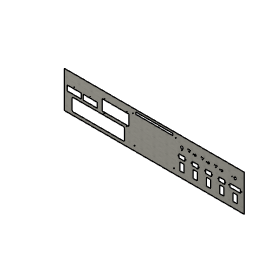
002_mounting_plate (Autodesk Fusion 360 design; units mm, degrees)
Autodesk Fusion 360 part; units mm, degrees
note: some values were not read from the file. Set by a fixed rule: the direction of a hole.
sketch "Sketch1" plane through (360, 70, -13) normal (0, 0, -1) x (1, 0, 0)
  line L0 (100, 7.5) -> (124, 7.5)
  line L1 (124, 7.5) -> (124, -7.5)
  line L2 (124, -7.5) -> (100, -7.5)
  line L3 (100, -7.5) -> (100, 7.5)
  circle A0 centre (274, -35) radius 3.5
  circle A1 centre (220, -35) radius 3.5
  circle A2 centre (220, 35) radius 6.5
  circle A3 centre (166, 35) radius 6.5
  circle A4 centre (112, 35) radius 6.5
  circle A5 centre (274, 35) radius 6.5
  circle A6 centre (328, 35) radius 6.5
  line L4 (-210, -3.5) -> (-105, -3.5) construction
  line L5 (-105, -3.5) -> (-105, -43.5) construction
  line L6 (-105, -43.5) -> (-210, -43.5) construction
  line L7 (-210, -43.5) -> (-210, -3.5) construction
  circle A7 centre (328, -35) radius 4.5
  arc A8 (-121, 55.5) -> (-126, 60.5) centre (-126, 55.5) ccw
  line L8 (-121, 55.5) -> (-121, 14.5)
  arc A9 (-126, 9.5) -> (-121, 14.5) centre (-126, 14.5) ccw
  line L9 (-126, 9.5) -> (-329, 9.5)
  arc A10 (-334, 14.5) -> (-329, 9.5) centre (-329, 14.5) ccw
  line L10 (-334, 14.5) -> (-334, 55.5)
  arc A11 (-329, 60.5) -> (-334, 55.5) centre (-329, 55.5) ccw
  line L11 (-329, 60.5) -> (-126, 60.5)
  circle A12 centre (166, -35) radius 3.5
  circle A13 centre (112, -35) radius 5
  line L12 (-360, 70) -> (-360, -70)
  line L13 (-360, -70) -> (360, -70)
  line L14 (360, -70) -> (360, 70)
  line L15 (360, 70) -> (-360, 70)
  line L16 (-333.4, -12.9) -> (-333.4, -4.4) construction
  line L17 (-297.4, -2.4) -> (-352.4, -2.4) construction
  line L18 (-352.4, -2.4) -> (-352.4, -50.4) construction
  line L19 (-352.4, -50.4) -> (-297.4, -50.4) construction
  line L20 (-297.4, -50.4) -> (-297.4, -2.4) construction
  line L21 (-316.4, -4.4) -> (-316.4, -12.9) construction
  line L22 (-333.4, -4.4) -> (-333.4, -12.9) construction
  line L23 (-316.4, -12.9) -> (-316.4, -4.4) construction
  line L24 (-268.6, -4.4) -> (-268.6, -12.9) construction
  line L25 (-251.6, -12.9) -> (-251.6, -4.4) construction
  line L26 (-251.6, -4.4) -> (-251.6, -12.9) construction
  line L27 (-268.6, -12.9) -> (-268.6, -4.4) construction
  line L28 (-232.6, -2.4) -> (-287.6, -2.4) construction
  line L29 (-287.6, -2.4) -> (-287.6, -50.4) construction
  line L30 (-287.6, -50.4) -> (-232.6, -50.4) construction
  line L31 (-232.6, -50.4) -> (-232.6, -2.4) construction
  line L32 (-231.6, -22.4) -> (-288.6, -22.4)
  line L33 (-288.6, -22.4) -> (-288.6, -1.4)
  line L34 (-288.6, -1.4) -> (-231.6, -1.4)
  line L35 (-231.6, -1.4) -> (-231.6, -22.4)
  line L36 (-287.6, -26.4) -> (-297.4, -26.4) construction
  line L37 (-292.5, -26.4) -> (-292.5, -42) construction
  line L38 (-353.4, -22.4) -> (-296.4, -22.4)
  line L39 (-353.4, -1.4) -> (-353.4, -22.4)
  line L40 (-296.4, -1.4) -> (-353.4, -1.4)
  line L41 (-296.4, -22.4) -> (-296.4, -1.4)
  line L42 (232, -7.5) -> (208, -7.5)
  line L43 (208, -7.5) -> (208, 7.5)
  line L44 (208, 7.5) -> (232, 7.5)
  line L45 (232, 7.5) -> (232, -7.5)
  line L46 (178, -7.5) -> (154, -7.5)
  line L47 (154, -7.5) -> (154, 7.5)
  line L48 (154, 7.5) -> (178, 7.5)
  line L49 (178, 7.5) -> (178, -7.5)
  line L50 (286, -7.5) -> (262, -7.5)
  line L51 (262, -7.5) -> (262, 7.5)
  line L52 (262, 7.5) -> (286, 7.5)
  line L53 (286, 7.5) -> (286, -7.5)
  circle A14 centre (328, 0) radius 4.6 construction
  circle A15 centre (343, 0) radius 4.6 construction
  circle A16 centre (313, 0) radius 4.6 construction
  line L54 (307, -7) -> (349, -7)
  line L55 (349, -7) -> (349, 7)
  line L56 (349, 7) -> (307, 7)
  line L57 (307, 7) -> (307, -7)
  line L58 (328, 0) -> (328, -7) construction
  line L59 (349, 0) -> (360, 0) construction
  circle A17 centre (353, 0) radius 1.6
  circle A18 centre (303, 0) radius 1.6
  line L60 (-360, 0) -> (360, 0) construction
  line L61 (0, -70) -> (0, 70) construction
  line L62 (-235, -43.5) -> (-285, -43.5) construction
  line L63 (-285, -43.5) -> (-285, -13.5) construction
  line L64 (-285, -13.5) -> (-235, -13.5) construction
  line L65 (-235, -13.5) -> (-235, -43.5) construction
  circle A19 centre (-260, -28.5) radius 2
  line L66 (-260, -43.5) -> (-260, -28.5) construction
  line L67 (-260, -28.5) -> (-235, -28.5) construction
  circle A20 centre (-325, -28.5) radius 2
  arc A21 (-333.4, -12.9) -> (-316.4, -12.9) centre (-324.9, -12.9) ccw
  line L68 (-333.4, -4.4) -> (-316.4, -4.4)
  line L69 (-316.4, -4.4) -> (-333.4, -4.4)
  arc A22 (-333.4, -12.9) -> (-316.4, -12.9) centre (-324.9, -12.9) ccw
  line L70 (-251.6, -4.4) -> (-268.6, -4.4)
  arc A23 (-268.6, -12.9) -> (-251.6, -12.9) centre (-260.1, -12.9) ccw
  line L71 (-268.6, -4.4) -> (-251.6, -4.4)
  arc A24 (-268.6, -12.9) -> (-251.6, -12.9) centre (-260.1, -12.9) ccw
  line L72 (-231.6, -21.4) -> (-288.6, -21.4) construction
  line L73 (365, 73) -> (-365, 73)
  line L74 (-365, 73) -> (-365, -75)
  line L75 (-365, -75) -> (365, -75)
  line L76 (365, -75) -> (365, 73)
  dimension "d326" = 42
  dimension "d327" = 14
  dimension "d330" = 3.2
  dimension "d331" = 7
  dimension "d334" = 4
  dimension "d811" = 4
  dimension "d819" = 1
  dimension "d820" = 1
  dimension "d821" = 1
  dimension "d822" = 1
  constraint horizontal L32
  constraint vertical L33
  constraint horizontal L34
  constraint vertical L35
  constraint midpoint L29 L36.start
  constraint midpoint L20 L36.end
  constraint midpoint L36 L37.start
  constraint perpendicular L36 L37
  constraint symmetric L32.start L37 L38.start
  constraint symmetric L32.end L37 L38.end
  constraint symmetric L33.end L37 L40.start
  constraint symmetric L34.end L37 L39.start
  constraint horizontal L54
  constraint vertical L55
  constraint horizontal L56
  constraint vertical L57
  constraint coincident A14.centre L58.start
  constraint midpoint L54 L58.end
  constraint vertical L58
  constraint midpoint L55 L59.start
  constraint midpoint L14 L59.end
  constraint horizontal L59
  constraint symmetric L58 A17 A18
  constraint midpoint L12 L60.start
  constraint midpoint L13 L61.start
  constraint midpoint L15 L61.end
  constraint midpoint L62 L66.start
  constraint coincident A19.centre L66.end
  constraint perpendicular L62 L66
  constraint midpoint L65 L67.end
  constraint perpendicular L65 L67
  constraint symmetric L37 A19 A20
  constraint coincident L35 L72.start
  constraint coincident L33 L72.end
  constraint perpendicular L33 L72
  constraint tangent A23 L72
  measures "d326" distance of L54.start L54.end
  measures "d327" distance of L54.start L56.end
  measures "d330" diameter of A17
  measures "d331" distance of L54 A17.centre
  measures "d334" distance of L55 A17.centre
  measures "d811" diameter of A19
  measures "d819" distance of L32 L72
  measures "d820" distance of L31 L35
  measures "d821" distance of L28 L34
  measures "d822" distance of L29 L33
extrude "Extrude1" add sketch "Sketch1" along normal blind 1 contours A2 | A3 | A4 | A5 | A6 | L12 L13 L14 L15 | A17 | A18 | A19 | A20
sketch "Sketch3" plane through (0, 0, -14) normal (0, 0, -1) x (-1, 0, 0)
  circle A0 centre (-580, 105) radius 3.5
  circle A1 centre (-634, 105) radius 3.5
  line L0 (-484, 77.5) -> (-460, 77.5)
  line L1 (-460, 77.5) -> (-460, 62.5)
  line L2 (-460, 62.5) -> (-484, 62.5)
  line L3 (-484, 62.5) -> (-484, 77.5)
  line L4 (-622, 62.5) -> (-646, 62.5)
  line L5 (-646, 62.5) -> (-646, 77.5)
  line L6 (-646, 77.5) -> (-622, 77.5)
  line L7 (-622, 77.5) -> (-622, 62.5)
  circle A2 centre (-688, 105) radius 4.5
  line L8 (-514, 62.5) -> (-538, 62.5)
  line L9 (-538, 62.5) -> (-538, 77.5)
  line L10 (-538, 77.5) -> (-514, 77.5)
  line L11 (-514, 77.5) -> (-514, 62.5)
  line L12 (-568, 62.5) -> (-592, 62.5)
  line L13 (-592, 62.5) -> (-592, 77.5)
  line L14 (-592, 77.5) -> (-568, 77.5)
  line L15 (-568, 77.5) -> (-568, 62.5)
  arc A3 (-26, 55.5) -> (-31, 60.5) centre (-31, 55.5) ccw
  line L16 (-26, 55.5) -> (-26, 14.5)
  arc A4 (-31, 9.5) -> (-26, 14.5) centre (-31, 14.5) ccw
  line L17 (-31, 9.5) -> (-234, 9.5)
  arc A5 (-239, 14.5) -> (-234, 9.5) centre (-234, 14.5) ccw construction
  line L18 (-239, 14.5) -> (-239, 55.5) construction
  arc A6 (-234, 60.5) -> (-239, 55.5) centre (-234, 55.5) ccw construction
  line L19 (-234, 60.5) -> (-31, 60.5)
  line L20 (-667, 77) -> (-667, 63)
  line L21 (-667, 63) -> (-709, 63)
  line L22 (-709, 63) -> (-709, 77)
  line L23 (-709, 77) -> (-667, 77)
  line L24 (-63.6, 71.4) -> (-63.6, 92.4)
  line L25 (-63.6, 92.4) -> (-6.6, 92.4)
  line L26 (-6.6, 92.4) -> (-6.6, 71.4)
  line L27 (-6.6, 71.4) -> (-63.6, 71.4)
  circle A7 centre (-526, 105) radius 3.5
  circle A8 centre (-472, 105) radius 5
  line L28 (-71.4, 71.4) -> (-128.4, 71.4)
  line L29 (-128.4, 71.4) -> (-128.4, 92.4)
  line L30 (-128.4, 92.4) -> (-71.4, 92.4)
  line L31 (-71.4, 92.4) -> (-71.4, 71.4)
  line L32 (-720, 0) -> (0, 0)
  line L33 (0, 0) -> (0, 140)
  line L34 (0, 140) -> (-720, 140)
  line L35 (-720, 140) -> (-720, 0)
  line L36 (-275, 17.5) -> (-275, 128.5) construction
  line L37 (-445, 17.5) -> (-275, 17.5) construction
  line L38 (-445, 128.5) -> (-445, 17.5) construction
  line L39 (-275, 128.5) -> (-445, 128.5) construction
  circle A9 centre (-447, 126.5) radius 1.5
  line L40 (-275, 73) -> (-445, 73) construction
  line L41 (-360, 17.5) -> (-360, 128.5) construction
  circle A10 centre (-273, 126.5) radius 1.5
  circle A11 centre (-440, 16) radius 1.5
  circle A12 centre (-280, 16) radius 1.5
  line L42 (-285, 128.5) -> (-435, 128.5)
  line L43 (-435, 128.5) -> (-435, 136.5)
  line L44 (-435, 136.5) -> (-285, 136.5)
  line L45 (-285, 136.5) -> (-285, 128.5)
  line L46 (-200, 114.5) -> (-200, 113.5) construction
  line L47 (-200, 113.5) -> (-205, 113.5) construction
  line L48 (-205, 113.5) -> (-205, 114.5) construction
  line L49 (-205, 114.5) -> (-255, 114.5) construction
  line L50 (-255, 114.5) -> (-255, 96) construction
  line L51 (-255, 96) -> (-256, 96) construction
  line L52 (-256, 96) -> (-256, 91) construction
  line L53 (-256, 91) -> (-255, 91) construction
  line L54 (-255, 91) -> (-255, 72.5) construction
  line L55 (-255, 72.5) -> (-205, 72.5) construction
  line L56 (-205, 72.5) -> (-205, 73.5) construction
  line L57 (-205, 73.5) -> (-200, 73.5) construction
  line L58 (-200, 73.5) -> (-200, 72.5) construction
  line L59 (-200, 72.5) -> (-150, 72.5) construction
  line L60 (-150, 72.5) -> (-150, 91) construction
  line L61 (-150, 96) -> (-150, 114.5) construction
  line L62 (-150, 114.5) -> (-200, 114.5) construction
  line L63 (-256.5, 115) -> (-148.5, 115)
  line L64 (-148.5, 115) -> (-148.5, 72)
  line L65 (-148.5, 72) -> (-256.5, 72)
  line L66 (-256.5, 72) -> (-256.5, 115)
  line L67 (-150, 91) -> (-149, 91)
  line L68 (-149, 91) -> (-149, 96)
  line L69 (-149, 96) -> (-150, 96)
  dimension "d480" = 3
  dimension "d483" = 150
  dimension "d484" = 8
  dimension "d491" = 5
  dimension "d492" = 2
  dimension "d493" = 2
  dimension "d801" = 0.5
  dimension "d802" = 0.5
  dimension "d803" = 0.5
  constraint midpoint L36 L40.start
  constraint midpoint L38 L40.end
  constraint midpoint L37 L41.start
  constraint midpoint L39 L41.end
  constraint symmetric A9 L41 A10
  constraint horizontal L42
  constraint vertical L43
  constraint horizontal L44
  constraint vertical L45
  constraint coincident L39 L42.start
  constraint symmetric L41 L43 L45
  constraint equal A9 A11
  constraint equal A11 A12
  constraint symmetric L41 A11 A12
  constraint tangent L37 A11
  constraint horizontal L63
  constraint vertical L64
  constraint horizontal L65
  constraint vertical L66
  measures "d480" diameter of A9
  measures "d483" distance of L43.end L44.end
  measures "d484" distance of L42.end L43.end
  measures "d491" distance of L38 A11.centre
  measures "d492" distance of L39 A9.centre
  measures "d493" distance of L38 A9.centre
  measures "d801" distance of L59 L65
  measures "d802" distance of L52 L66
  measures "d803" distance of L49 L63
extrude "Extrude4" cut sketch "Sketch3" against normal up to surface (1 mm away) contours L42 L43 L44 L45 | L63 L64 L65 L66
hole "Hole1" at (447, 126.5, -14) at (440, 16, -14) at (280, 16, -14) at (273, 126.5, -14) direction (0, 0, 1) diameter 3.4 depth 2 tip angle 118
sketch "Sketch4" plane through (360, 70, -5) normal (0, 0, 1) x (1, 0, 0)
  circle A0 centre (146.55, 41.35) radius 1 construction
  circle A1 centre (141.55, 41.35) radius 1 construction
  circle A2 centre (136.55, 41.35) radius 1 construction
  circle A3 centre (141.55, 35) radius 1.5
  circle A4 centre (136.55, 41.35) radius 1.2
  circle A5 centre (141.55, 41.35) radius 1.2
  circle A6 centre (146.55, 41.35) radius 1.2
  circle A7 centre (141.55, 35) radius 1.6
  line L0 (158.5, 33.6282) -> (158.5, 36.2282) construction
  line L1 (158.5, 36.2282) -> (157.5, 36.2282) construction
  line L2 (157.5, 36.2282) -> (157.5, 33.6282) construction
  line L3 (157.5, 33.6282) -> (158.5, 33.6282) construction
  line L4 (157.3, 33.4282) -> (158.7, 33.4282)
  line L5 (158.7, 33.4282) -> (158.7, 36.4282)
  line L6 (158.7, 36.4282) -> (157.3, 36.4282)
  line L7 (157.3, 36.4282) -> (157.3, 33.4282)
  dimension "d578" = 0.2
  dimension "d579" = 0.2
  dimension "d580" = 0.2
  dimension "d581" = 3.2
  dimension "d628" = 0.2
  constraint concentric A3 A7
  measures "d581" diameter of A7
extrude "Extrude6" cut sketch "Sketch4" against normal up to surface (9 mm away) contours A5 | L4 L5 L6 L7
pattern_linear "R-Pattern1" count 3 spacing 54 along (1, 0, 0) of "Extrude6"
sketch "Sketch5" plane through (0, 0, -13) normal (0, 0, 1) x (1, 0, 0)
  circle A0 centre (609.55, 111.35) radius 1.2
  line L0 (625.3, 106.4282) -> (626.7, 106.4282)
  line L1 (626.7, 106.4282) -> (626.7, 103.4282)
  line L2 (626.7, 103.4282) -> (625.3, 103.4282)
  line L3 (625.3, 103.4282) -> (625.3, 106.4282)
  circle A1 centre (555.55, 111.35) radius 1.2
  line L4 (571.3, 106.4282) -> (572.7, 106.4282)
  line L5 (572.7, 106.4282) -> (572.7, 103.4282)
  line L6 (572.7, 103.4282) -> (571.3, 103.4282)
  line L7 (571.3, 103.4282) -> (571.3, 106.4282)
  circle A2 centre (501.55, 111.35) radius 1.2
  line L8 (517.3, 106.4282) -> (518.7, 106.4282)
  line L9 (518.7, 106.4282) -> (518.7, 103.4282)
  line L10 (518.7, 103.4282) -> (517.3, 103.4282)
  line L11 (517.3, 103.4282) -> (517.3, 106.4282)
  circle A3 centre (280, 16) radius 1.7
  circle A4 centre (447, 126.5) radius 1.7
  circle A5 centre (440, 16) radius 1.7
  circle A6 centre (273, 126.5) radius 1.7
  line L12 (285, 128.5) -> (285, 136.5)
  line L13 (285, 136.5) -> (435, 136.5)
  line L14 (435, 136.5) -> (435, 128.5)
  line L15 (435, 128.5) -> (285, 128.5)
  circle A7 centre (688, 105) radius 4.5
  arc A8 (31, 60.5) -> (26, 55.5) centre (31, 55.5) ccw
  line L16 (31, 60.5) -> (234, 60.5)
  arc A9 (239, 55.5) -> (234, 60.5) centre (234, 55.5) ccw
  line L17 (239, 55.5) -> (239, 14.5)
  arc A10 (234, 9.5) -> (239, 14.5) centre (234, 14.5) ccw
  line L18 (234, 9.5) -> (31, 9.5)
  arc A11 (26, 14.5) -> (31, 9.5) centre (31, 14.5) ccw
  line L19 (26, 14.5) -> (26, 55.5)
  line L20 (667, 63) -> (667, 77)
  line L21 (667, 77) -> (709, 77)
  line L22 (709, 77) -> (709, 63)
  line L23 (709, 63) -> (667, 63)
  line L24 (460, 77.5) -> (484, 77.5)
  line L25 (484, 77.5) -> (484, 62.5)
  line L26 (484, 62.5) -> (460, 62.5)
  line L27 (460, 62.5) -> (460, 77.5)
  line L28 (592, 62.5) -> (568, 62.5)
  line L29 (568, 62.5) -> (568, 77.5)
  line L30 (568, 77.5) -> (592, 77.5)
  line L31 (592, 77.5) -> (592, 62.5)
  circle A12 centre (580, 105) radius 3.5
  line L32 (646, 62.5) -> (622, 62.5)
  line L33 (622, 62.5) -> (622, 77.5)
  line L34 (622, 77.5) -> (646, 77.5)
  line L35 (646, 77.5) -> (646, 62.5)
  line L36 (63.6, 92.4) -> (63.6, 71.4)
  line L37 (63.6, 71.4) -> (6.6, 71.4)
  line L38 (6.6, 71.4) -> (6.6, 92.4)
  line L39 (6.6, 92.4) -> (63.6, 92.4)
  line L40 (538, 62.5) -> (514, 62.5)
  line L41 (514, 62.5) -> (514, 77.5)
  line L42 (514, 77.5) -> (538, 77.5)
  line L43 (538, 77.5) -> (538, 62.5)
  line L44 (128.4, 71.4) -> (71.4, 71.4)
  line L45 (71.4, 71.4) -> (71.4, 92.4)
  line L46 (71.4, 92.4) -> (128.4, 92.4)
  line L47 (128.4, 92.4) -> (128.4, 71.4)
  circle A13 centre (634, 105) radius 3.5
  circle A14 centre (472, 105) radius 5
  circle A15 centre (526, 105) radius 3.5
  line L48 (0, 0) -> (720, 0)
  line L49 (720, 0) -> (720, 140)
  line L50 (720, 140) -> (0, 140)
  line L51 (0, 140) -> (0, 0)
  circle A16 centre (457.625, 70) radius 1.5 construction
  circle A17 centre (486.375, 70) radius 1.5 construction
  circle A18 centre (457.625, 70) radius 1.7
  circle A19 centre (486.375, 70) radius 1.7
  line L52 (256.5, 115) -> (256.5, 72)
  line L53 (256.5, 72) -> (148.5, 72)
  line L54 (148.5, 72) -> (148.5, 115)
  line L55 (148.5, 115) -> (256.5, 115)
  dimension "d648" = 0.2
  constraint concentric A17 A19
  constraint equal A18 A19
sketch "Sketch6" plane through (0, 0, -13) normal (0, 0, 1) x (1, 0, 0)
  circle A0 centre (609.55, 111.35) radius 1.2
  line L0 (625.3, 106.4282) -> (626.7, 106.4282)
  line L1 (626.7, 106.4282) -> (626.7, 103.4282)
  line L2 (626.7, 103.4282) -> (625.3, 103.4282)
  line L3 (625.3, 103.4282) -> (625.3, 106.4282)
  circle A1 centre (555.55, 111.35) radius 1.2
  line L4 (571.3, 106.4282) -> (572.7, 106.4282)
  line L5 (572.7, 106.4282) -> (572.7, 103.4282)
  line L6 (572.7, 103.4282) -> (571.3, 103.4282)
  line L7 (571.3, 103.4282) -> (571.3, 106.4282)
  circle A2 centre (501.55, 111.35) radius 1.2
  line L8 (517.3, 106.4282) -> (518.7, 106.4282)
  line L9 (518.7, 106.4282) -> (518.7, 103.4282)
  line L10 (518.7, 103.4282) -> (517.3, 103.4282)
  line L11 (517.3, 103.4282) -> (517.3, 106.4282)
  circle A3 centre (280, 16) radius 1.7
  circle A4 centre (447, 126.5) radius 1.7
  circle A5 centre (440, 16) radius 1.7
  circle A6 centre (273, 126.5) radius 1.7
  line L12 (285, 128.5) -> (285, 136.5)
  line L13 (285, 136.5) -> (435, 136.5)
  line L14 (435, 136.5) -> (435, 128.5)
  line L15 (435, 128.5) -> (285, 128.5)
  line L16 (667, 63) -> (667, 77)
  line L17 (667, 77) -> (709, 77)
  line L18 (709, 77) -> (709, 63)
  line L19 (709, 63) -> (667, 63)
  circle A7 centre (634, 105) radius 3.5
  circle A8 centre (580, 105) radius 3.5
  line L20 (646, 62.5) -> (622, 62.5)
  line L21 (622, 62.5) -> (622, 77.5)
  line L22 (622, 77.5) -> (646, 77.5)
  line L23 (646, 77.5) -> (646, 62.5)
  line L24 (460, 77.5) -> (484, 77.5)
  line L25 (484, 77.5) -> (484, 62.5)
  line L26 (484, 62.5) -> (460, 62.5)
  line L27 (460, 62.5) -> (460, 77.5)
  line L28 (538, 62.5) -> (514, 62.5)
  line L29 (514, 62.5) -> (514, 77.5)
  line L30 (514, 77.5) -> (538, 77.5)
  line L31 (538, 77.5) -> (538, 62.5)
  line L32 (592, 62.5) -> (568, 62.5)
  line L33 (568, 62.5) -> (568, 77.5)
  line L34 (568, 77.5) -> (592, 77.5)
  line L35 (592, 77.5) -> (592, 62.5)
  line L36 (63.6, 92.4) -> (63.6, 71.4)
  line L37 (63.6, 71.4) -> (6.6, 71.4)
  line L38 (6.6, 71.4) -> (6.6, 92.4)
  line L39 (6.6, 92.4) -> (63.6, 92.4)
  circle A9 centre (526, 105) radius 3.5
  circle A10 centre (472, 105) radius 5
  line L40 (128.4, 71.4) -> (71.4, 71.4)
  line L41 (71.4, 71.4) -> (71.4, 92.4)
  line L42 (71.4, 92.4) -> (128.4, 92.4)
  line L43 (128.4, 92.4) -> (128.4, 71.4)
  arc A11 (31, 60.5) -> (26, 55.5) centre (31, 55.5) ccw
  line L44 (31, 60.5) -> (234, 60.5)
  arc A12 (239, 55.5) -> (234, 60.5) centre (234, 55.5) ccw
  line L45 (239, 55.5) -> (239, 14.5)
  arc A13 (234, 9.5) -> (239, 14.5) centre (234, 14.5) ccw
  line L46 (234, 9.5) -> (31, 9.5)
  arc A14 (26, 14.5) -> (31, 9.5) centre (31, 14.5) ccw
  line L47 (26, 14.5) -> (26, 55.5)
  circle A15 centre (688, 105) radius 4.5 construction
  line L48 (0, 0) -> (720, 0)
  line L49 (720, 0) -> (720, 140)
  line L50 (720, 140) -> (0, 140)
  line L51 (0, 140) -> (0, 0)
  line L52 (701, 87) -> (675, 87) construction
  line L53 (675, 87) -> (675, 117) construction
  line L54 (675, 117) -> (701, 117) construction
  line L55 (701, 117) -> (701, 87) construction
  circle A16 centre (688, 105) radius 4.4
  line L56 (675, 106.3) -> (675.5, 106.3) construction
  line L57 (675.5, 106.3) -> (675.5, 103.7) construction
  line L58 (675.5, 103.7) -> (675, 103.7) construction
  line L59 (675, 103.7) -> (675, 106.3) construction
  line L60 (688, 105) -> (675.5, 105) construction
  line L61 (675.7, 103.5) -> (674.8, 103.5)
  line L62 (674.8, 103.5) -> (674.8, 106.5)
  line L63 (674.8, 106.5) -> (675.7, 106.5)
  line L64 (675.7, 106.5) -> (675.7, 103.5)
  line L65 (256.5, 115) -> (256.5, 72)
  line L66 (256.5, 72) -> (148.5, 72)
  line L67 (148.5, 72) -> (148.5, 115)
  line L68 (148.5, 115) -> (256.5, 115)
  dimension "d643" = 0.5
  dimension "d644" = 2.6
  dimension "d645" = -0.2
  constraint horizontal L56
  constraint vertical L57
  constraint horizontal L58
  constraint vertical L59
  constraint coincident A15.centre A16.centre
  constraint midpoint L57 L60.end
  constraint horizontal L60
  constraint collinear L53 L59
  measures "d643" distance of L56.start L56.end
  measures "d644" distance of L56.start L58.end
extrude "Extrude8" cut sketch "Sketch6" against normal up to surface (1 mm away) contours L61 L62 L63 L64
sketch "Sketch7" plane through (0, 0, -13) normal (0, 0, 1) x (1, 0, 0)
  line L0 (675.7, 106.5) -> (675.7, 103.5)
  line L1 (675.7, 103.5) -> (674.8, 103.5)
  line L2 (674.8, 103.5) -> (674.8, 106.5)
  line L3 (674.8, 106.5) -> (675.7, 106.5)
  circle A0 centre (609.55, 111.35) radius 1.2
  line L4 (625.3, 106.4282) -> (626.7, 106.4282)
  line L5 (626.7, 106.4282) -> (626.7, 103.4282)
  line L6 (626.7, 103.4282) -> (625.3, 103.4282)
  line L7 (625.3, 103.4282) -> (625.3, 106.4282)
  circle A1 centre (555.55, 111.35) radius 1.2
  line L8 (571.3, 106.4282) -> (572.7, 106.4282)
  line L9 (572.7, 106.4282) -> (572.7, 103.4282)
  line L10 (572.7, 103.4282) -> (571.3, 103.4282)
  line L11 (571.3, 103.4282) -> (571.3, 106.4282)
  circle A2 centre (501.55, 111.35) radius 1.2
  line L12 (517.3, 106.4282) -> (518.7, 106.4282)
  line L13 (518.7, 106.4282) -> (518.7, 103.4282)
  line L14 (518.7, 103.4282) -> (517.3, 103.4282)
  line L15 (517.3, 103.4282) -> (517.3, 106.4282)
  circle A3 centre (280, 16) radius 1.7
  circle A4 centre (447, 126.5) radius 1.7
  circle A5 centre (440, 16) radius 1.7
  circle A6 centre (273, 126.5) radius 1.7
  line L16 (285, 128.5) -> (285, 136.5)
  line L17 (285, 136.5) -> (435, 136.5)
  line L18 (435, 136.5) -> (435, 128.5)
  line L19 (435, 128.5) -> (285, 128.5)
  line L20 (63.6, 92.4) -> (63.6, 71.4)
  line L21 (63.6, 71.4) -> (6.6, 71.4)
  line L22 (6.6, 71.4) -> (6.6, 92.4)
  line L23 (6.6, 92.4) -> (63.6, 92.4)
  line L24 (667, 63) -> (667, 77)
  line L25 (667, 77) -> (709, 77)
  line L26 (709, 77) -> (709, 63)
  line L27 (709, 63) -> (667, 63)
  circle A7 centre (634, 105) radius 3.5
  circle A8 centre (580, 105) radius 3.5
  line L28 (646, 62.5) -> (622, 62.5)
  line L29 (622, 62.5) -> (622, 77.5)
  line L30 (622, 77.5) -> (646, 77.5)
  line L31 (646, 77.5) -> (646, 62.5)
  line L32 (592, 62.5) -> (568, 62.5)
  line L33 (568, 62.5) -> (568, 77.5)
  line L34 (568, 77.5) -> (592, 77.5)
  line L35 (592, 77.5) -> (592, 62.5)
  line L36 (538, 62.5) -> (514, 62.5)
  line L37 (514, 62.5) -> (514, 77.5)
  line L38 (514, 77.5) -> (538, 77.5)
  line L39 (538, 77.5) -> (538, 62.5)
  line L40 (128.4, 71.4) -> (71.4, 71.4)
  line L41 (71.4, 71.4) -> (71.4, 92.4)
  line L42 (71.4, 92.4) -> (128.4, 92.4)
  line L43 (128.4, 92.4) -> (128.4, 71.4)
  circle A9 centre (472, 105) radius 5
  circle A10 centre (526, 105) radius 3.5
  line L44 (460, 77.5) -> (484, 77.5)
  line L45 (484, 77.5) -> (484, 62.5)
  line L46 (484, 62.5) -> (460, 62.5)
  line L47 (460, 62.5) -> (460, 77.5)
  arc A11 (31, 60.5) -> (26, 55.5) centre (31, 55.5) ccw
  line L48 (31, 60.5) -> (234, 60.5)
  arc A12 (239, 55.5) -> (234, 60.5) centre (234, 55.5) ccw
  line L49 (239, 55.5) -> (239, 14.5)
  arc A13 (234, 9.5) -> (239, 14.5) centre (234, 14.5) ccw
  line L50 (234, 9.5) -> (31, 9.5)
  arc A14 (26, 14.5) -> (31, 9.5) centre (31, 14.5) ccw
  line L51 (26, 14.5) -> (26, 55.5)
  circle A15 centre (688, 105) radius 4.5
  line L52 (0, 0) -> (720, 0)
  line L53 (720, 0) -> (720, 140)
  line L54 (720, 140) -> (0, 140)
  line L55 (0, 140) -> (0, 0)
  line L56 (468.75, 21) -> (475.25, 21) construction
  line L57 (475.25, 21) -> (475.25, 22) construction
  line L58 (475.25, 22) -> (468.75, 22) construction
  line L59 (468.75, 22) -> (468.75, 21) construction
  line L60 (475.25, 48) -> (475.25, 49) construction
  line L61 (475.25, 49) -> (468.75, 49) construction
  line L62 (468.75, 49) -> (468.75, 48) construction
  line L63 (468.75, 48) -> (475.25, 48) construction
  line L64 (480, 20) -> (464, 20) construction
  line L65 (464, 20) -> (464, 50) construction
  line L66 (464, 50) -> (480, 50) construction
  line L67 (480, 50) -> (480, 20) construction
  line L68 (480.5, 19.5) -> (463.5, 19.5)
  line L69 (463.5, 19.5) -> (463.5, 50.5)
  line L70 (463.5, 50.5) -> (480.5, 50.5)
  line L71 (480.5, 50.5) -> (480.5, 19.5)
  line L72 (256.5, 115) -> (256.5, 72)
  line L73 (256.5, 72) -> (148.5, 72)
  line L74 (148.5, 72) -> (148.5, 115)
  line L75 (148.5, 115) -> (256.5, 115)
  dimension "d649" = -0.5
extrude "Extrude9" cut sketch "Sketch7" against normal up to surface (1 mm away) contours L68 L69 L70 L71
pattern_linear "R-Pattern3" count 5 spacing 54 along (1, 0, 0) of "Extrude9"
sketch "Sketch9" plane through (0, 0, -14) normal (0, 0, -1) x (-1, 0, 0)
  line L0 (-696.5, 19.5) -> (-696.5, 50.5)
  line L1 (-696.5, 50.5) -> (-679.5, 50.5)
  line L2 (-679.5, 50.5) -> (-679.5, 19.5)
  line L3 (-679.5, 19.5) -> (-696.5, 19.5)
  line L4 (-642.5, 19.5) -> (-642.5, 50.5)
  line L5 (-642.5, 50.5) -> (-625.5, 50.5)
  line L6 (-625.5, 50.5) -> (-625.5, 19.5)
  line L7 (-625.5, 19.5) -> (-642.5, 19.5)
  line L8 (-588.5, 19.5) -> (-588.5, 50.5)
  line L9 (-588.5, 50.5) -> (-571.5, 50.5)
  line L10 (-571.5, 50.5) -> (-571.5, 19.5)
  line L11 (-571.5, 19.5) -> (-588.5, 19.5)
  line L12 (-534.5, 19.5) -> (-534.5, 50.5)
  line L13 (-534.5, 50.5) -> (-517.5, 50.5)
  line L14 (-517.5, 50.5) -> (-517.5, 19.5)
  line L15 (-517.5, 19.5) -> (-534.5, 19.5)
  line L16 (-480.5, 19.5) -> (-480.5, 50.5)
  line L17 (-480.5, 50.5) -> (-463.5, 50.5)
  line L18 (-463.5, 50.5) -> (-463.5, 19.5)
  line L19 (-463.5, 19.5) -> (-480.5, 19.5)
  line L20 (-675.7, 103.5) -> (-675.7, 106.5)
  line L21 (-675.7, 106.5) -> (-674.8, 106.5)
  line L22 (-674.8, 106.5) -> (-674.8, 103.5)
  line L23 (-674.8, 103.5) -> (-675.7, 103.5)
  circle A0 centre (-609.55, 111.35) radius 1.2
  line L24 (-626.7, 106.4282) -> (-625.3, 106.4282)
  line L25 (-625.3, 106.4282) -> (-625.3, 103.4282)
  line L26 (-625.3, 103.4282) -> (-626.7, 103.4282)
  line L27 (-626.7, 103.4282) -> (-626.7, 106.4282)
  circle A1 centre (-555.55, 111.35) radius 1.2
  line L28 (-572.7, 106.4282) -> (-571.3, 106.4282)
  line L29 (-571.3, 106.4282) -> (-571.3, 103.4282)
  line L30 (-571.3, 103.4282) -> (-572.7, 103.4282)
  line L31 (-572.7, 103.4282) -> (-572.7, 106.4282)
  circle A2 centre (-501.55, 111.35) radius 1.2
  line L32 (-518.7, 106.4282) -> (-517.3, 106.4282)
  line L33 (-517.3, 106.4282) -> (-517.3, 103.4282)
  line L34 (-517.3, 103.4282) -> (-518.7, 103.4282)
  line L35 (-518.7, 103.4282) -> (-518.7, 106.4282)
  circle A3 centre (-280, 16) radius 1.7
  circle A4 centre (-447, 126.5) radius 1.7
  circle A5 centre (-440, 16) radius 1.7
  circle A6 centre (-273, 126.5) radius 1.7
  line L36 (-285, 136.5) -> (-285, 128.5)
  line L37 (-285, 128.5) -> (-435, 128.5)
  line L38 (-435, 128.5) -> (-435, 136.5)
  line L39 (-435, 136.5) -> (-285, 136.5)
  line L40 (-256.5, 72) -> (-256.5, 115) construction
  line L41 (-256.5, 115) -> (-148.5, 115) construction
  line L42 (-148.5, 115) -> (-148.5, 72) construction
  line L43 (-148.5, 72) -> (-256.5, 72) construction
  line L44 (-568, 62.5) -> (-592, 62.5)
  line L45 (-592, 62.5) -> (-592, 77.5)
  line L46 (-592, 77.5) -> (-568, 77.5)
  line L47 (-568, 77.5) -> (-568, 62.5)
  circle A7 centre (-472, 105) radius 5
  line L48 (-63.6, 71.4) -> (-63.6, 92.4)
  line L49 (-63.6, 92.4) -> (-6.6, 92.4)
  line L50 (-6.6, 92.4) -> (-6.6, 71.4)
  line L51 (-6.6, 71.4) -> (-63.6, 71.4)
  line L52 (-484, 77.5) -> (-460, 77.5)
  line L53 (-460, 77.5) -> (-460, 62.5)
  line L54 (-460, 62.5) -> (-484, 62.5)
  line L55 (-484, 62.5) -> (-484, 77.5)
  line L56 (-667, 77) -> (-667, 63)
  line L57 (-667, 63) -> (-709, 63)
  line L58 (-709, 63) -> (-709, 77)
  line L59 (-709, 77) -> (-667, 77)
  circle A8 centre (-634, 105) radius 3.5
  line L60 (-622, 62.5) -> (-646, 62.5)
  line L61 (-646, 62.5) -> (-646, 77.5)
  line L62 (-646, 77.5) -> (-622, 77.5)
  line L63 (-622, 77.5) -> (-622, 62.5)
  circle A9 centre (-526, 105) radius 3.5
  circle A10 centre (-580, 105) radius 3.5
  arc A11 (-26, 55.5) -> (-31, 60.5) centre (-31, 55.5) ccw
  line L64 (-26, 55.5) -> (-26, 14.5)
  arc A12 (-31, 9.5) -> (-26, 14.5) centre (-31, 14.5) ccw
  line L65 (-31, 9.5) -> (-234, 9.5)
  arc A13 (-239, 14.5) -> (-234, 9.5) centre (-234, 14.5) ccw
  line L66 (-239, 14.5) -> (-239, 55.5)
  arc A14 (-234, 60.5) -> (-239, 55.5) centre (-234, 55.5) ccw
  line L67 (-234, 60.5) -> (-31, 60.5)
  line L68 (-514, 62.5) -> (-538, 62.5)
  line L69 (-538, 62.5) -> (-538, 77.5)
  line L70 (-538, 77.5) -> (-514, 77.5)
  line L71 (-514, 77.5) -> (-514, 62.5)
  circle A15 centre (-688, 105) radius 4.5
  line L72 (-71.4, 71.4) -> (-128.4, 71.4)
  line L73 (-128.4, 71.4) -> (-128.4, 92.4)
  line L74 (-128.4, 92.4) -> (-71.4, 92.4)
  line L75 (-71.4, 92.4) -> (-71.4, 71.4)
  line L76 (-720, 0) -> (0, 0)
  line L77 (0, 0) -> (0, 140)
  line L78 (0, 140) -> (-720, 140)
  line L79 (-720, 140) -> (-720, 0)
  circle A16 centre (-248, 118.5) radius 2.5 construction
  circle A17 centre (-248, 93.5) radius 2.5 construction
  circle A18 centre (-248, 68.5) radius 2.5 construction
  line L80 (-258, 131) -> (-258, 61) construction
  line L81 (-258, 61) -> (-238, 61) construction
  line L82 (-238, 61) -> (-238, 131) construction
  line L83 (-238, 131) -> (-258, 131) construction
  circle A19 centre (-157, 118.5) radius 2.5 construction
  circle A20 centre (-157, 93.5) radius 2.5 construction
  circle A21 centre (-157, 68.5) radius 2.5 construction
  line L84 (-147, 61) -> (-147, 131) construction
  line L85 (-147, 131) -> (-167, 131) construction
  line L86 (-167, 131) -> (-167, 61) construction
  line L87 (-167, 61) -> (-147, 61) construction
  circle A22 centre (-248, 118.5) radius 2
  circle A23 centre (-157, 118.5) radius 2
  circle A24 centre (-157, 68.5) radius 2
  circle A25 centre (-248, 68.5) radius 2
  dimension "d739" = -0.5
  dimension "d740" = -0.5
  dimension "d741" = -0.5
  dimension "d742" = -0.5
hole "Hole2" at (100, 98.5, -13) at (35, 98.5, -13) direction (0, 0, -1) diameter 2.4 depth 1 tip angle 118
hole "Hole3" at (248, 118.5, -14) at (157, 118.5, -14) at (157, 68.5, -14) at (248, 68.5, -14) direction (0, 0, 1) diameter 3.4 depth 1 tip angle 118
hole "Hole4" at (496.55, 111.35, -5) at (506.55, 111.35, -5) direction (0, 0, -1) diameter 2.4 depth 9 tip angle 118
hole "Hole5" at (501.55, 105, -5) direction (0, 0, -1) diameter 3.4 depth 9 tip angle 118
pattern_linear "R-Pattern4" count 3 spacing 54 along (1, 0, 0) of "Hole4", "Hole5"
hole "Hole6" at (713, 70, -13) at (663, 70, -13) direction (0, 0, -1) diameter 3.4 depth 1 tip angle 118
hole "Hole7" at (486.375, 70, -13) at (457.625, 70, -13) direction (0, 0, -1) diameter 3.4 depth 1 tip angle 118
pattern_linear "R-Pattern5" count 4 spacing 54 along (1, 0, 0) of "Hole7"
extrude "Extrude13" add sketch "Sketch1" along normal up to surface (1 mm away) contours L73 L74 L75 L76
extrude "Extrude14" [suppressed]
sketch "Sketch11" plane through (360, 70, -13) normal (0, 0, -1) x (1, 0, 0)
  circle A0 centre (112, -35) radius 13
  circle A1 centre (112, -35) radius 5
  line L0 (112, -35) -> (112, -22) construction
  circle A2 centre (112, -25.75) radius 1.75
  dimension "d981" = 3.5
  dimension "d982" = 3.75
  constraint coincident A0.centre A1.centre
  constraint coincident A0 L0.end
  constraint vertical L0
  constraint coincident L0 A2.centre
  measures "d981" diameter of A2
  measures "d982" distance of L0.end A2.centre
hole "Hole8" at (472, 95.75, -13) direction (0, 0, -1) diameter 3.332 depth 1 tip angle 180
equation "d493 = d480 / 2 + 0.5 mm"
equation "d645 = 0 mm - 0.2 mm"
equation "d740 = d739"
equation "d741 = d739"
equation "d742 = d739"
equation "d801 = d800"
equation "d802 = d800"
equation "d803 = d800"
equation "d820 = d819"
equation "d821 = d819"
equation "d822 = d819"
equation "d982 = d981 / 2 + 2 mm"
equation "d800 = 0.5 mm"
